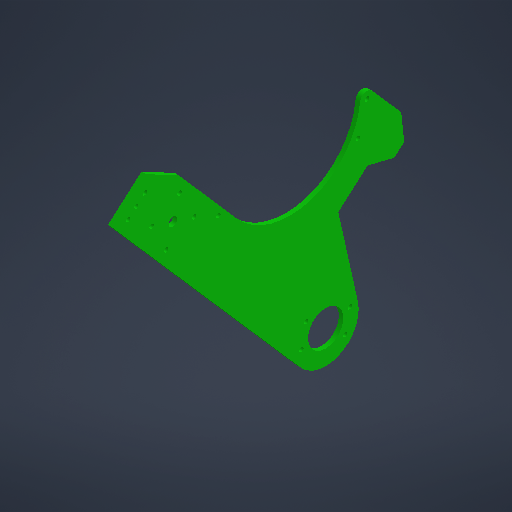
# Autodesk Inventor part: CHAPA LATERAL INTAKE V2
Saved by Autodesk Inventor 2026 (Build 300175000, 175)
## iProperties
Created: 2026-06-24
Part Number: CHAPA LATERAL INTAKE V2
Material: Genérico
Document SubType Name: Modeling
Designer: DELL
Density: 1 g/cm^3
Appearance: Verde escuro
Author: DELL
Autodesk Inventor part; units mm, degrees
ref_plane "YZ Plane" through (0, 0, 0) normal (1, 0, 0) x (0, 1, 0)
ref_plane "XZ Plane" through (0, 0, 0) normal (0, 1, 0) x (-1, 0, 0)
ref_plane "XY Plane" through (0, 0, 0) normal (0, 0, 1) x (1, 0, 0)
sketch "Esboço1" plane through (0, 0, 0) normal (1, 0, 0) x (0, 1, 0)
  circle A0 centre (0, 0) radius 20
  circle A1 centre (0, 0) radius 37.5
  dimension "d0" = 40
  dimension "d1" = 75
  constraints: 2 centre point, 2 coincident
  measures "d0" diameter of A0
  measures "d1" diameter of A1
extrude "Extrusão1" add sketch "Esboço1" along normal blind 5
sketch "Esboço3" plane through (5, 0, 0) normal (1, 0, 0) x (0, 0, -1)
  line L0 (154.1962, 109.7603) -> (153.014, 111.1125) projected
  line L1 (40.5387, 95.9825) -> (78.7824, 129.4199) projected
  line L2 (153.014, 111.1125) -> (-99.3237, 399.7205)
  circle A0 centre (0, 0) radius 37.5 projected
  line L3 (-28.231, -24.6832) -> (-242.5302, 220.4188)
  arc A1 (-100.8216, 158.3529) -> (38.988, 202.8563) centre (-40.5953, 211.0103) ccw
  line L4 (-100.8216, 158.3529) -> (-166.6433, 233.6357)
  line L5 (-166.6433, 233.6357) -> (-204.2865, 253.8562)
  circle A2 centre (46.9464, 202.0409) radius 2.5
  circle A3 centre (36.4428, 168.4765) radius 2.5
  arc A4 (52.969, 207.3066) -> (38.988, 202.8563) centre (46.9464, 202.0409) ccw
  line L6 (52.969, 207.3066) -> (85.8799, 169.6652)
  line L7 (85.8799, 169.6652) -> (14.3612, 107.1346)
  line L8 (14.3612, 107.1346) -> (36.5877, 8.2215)
  circle A5 centre (-224.6099, 219.2172) radius 2.5
  circle A6 centre (-205.4881, 235.936) radius 2.5
  circle A7 centre (-215.049, 227.5766) radius 2.5
  line L9 (-242.5302, 220.4188) -> (-204.2865, 253.8562)
  dimension "d5" = 160
  dimension "d10" = 100
  dimension "d11" = 5
  dimension "d12" = 5
  dimension "d13" = 88
  dimension "d14" = 88
  dimension "d15" = 20
  dimension "d16" = 50
  dimension "d18" = 50
  dimension "d19" = 95
  dimension "d20" = 5
  dimension "d21" = 5
  dimension "d22" = 5
  dimension "d23" = 12.7
  dimension "d25" = 12.7
  dimension "d30" = 280
  dimension "d31" = 140
  dimension "d32" = 12.7
  dimension "d33" = 12.7
  dimension "d34" = 12.7
  dimension "d35" = 12.7
  constraints: 16 end point, 7 centre point, 7 point on circle, 6 tangent, 3 perpendicular, 1 coincident, 1 point on line
  measures "d5" diameter of A1
  measures "d10" distance of L4.start L4.end
  measures "d11" diameter of A2
  measures "d12" diameter of A3
  measures "d13" distance of A1.centre A2.centre
  measures "d14" distance of A1.centre A3.centre
  measures "d15" distance from line of L2 A2.centre
  measures "d16" distance from line of L2 A3.centre
  measures "d18" distance of L6.start L6.end
  measures "d19" distance of L6.end L7.end
  measures "d20" diameter of A5
  measures "d21" diameter of A6
  measures "d22" diameter of A7
  measures "d23" distance of A5.centre A7.centre
  measures "d25" distance of A6.centre A7.centre
  measures "d30" distance between parallel lines of L1 L9
  measures "d31" distance from line of L9 A1.centre
  measures "d32" distance from line of L9 A5.centre
  measures "d33" distance from line of L9 A7.centre
  measures "d34" distance from line of L9 A6.centre
  measures "d35" distance from line of L3 A5.centre
extrude "Extrusão2" add sketch "Esboço3" against normal blind 5 contours A0 L3 L9 L5 L4 A1 A4 L6 L7 L8
sketch "Esboço4" plane through (5, 0, 0) normal (1, 0, 0) x (0, 0, -1)
  line L0 (154.1962, 109.7603) -> (153.014, 111.1125) projected
  line L1 (153.014, 111.1125) -> (-112.9577, 415.3142)
  circle A0 centre (-34.8401, 212.0241) radius 75
  circle A1 centre (-121.7601, 171.9256) radius 20
  line L2 (-204.2865, 253.8562) -> (-242.5302, 220.4188) projected
  line L3 (-242.5302, 220.4188) -> (-28.231, -24.6832) projected
  circle A2 centre (-121.7601, 171.9256) radius 2.5
  circle A3 centre (-173.5863, 191.7005) radius 5
  circle A4 centre (-22.3357, 17.5375) radius 2.5 projected
  circle A5 centre (-27.4315, -7.3461) radius 2.5 projected
  circle A6 centre (22.3357, -17.5375) radius 2.5 projected
  circle A7 centre (27.4315, 7.3461) radius 2.5 projected
  point P0 (0, 0)
  dimension "d38" = 150
  dimension "d39" = 40
  dimension "d40" = 116
  dimension "d41" = 59
  dimension "d42" = 5
  dimension "d43" = 10
  dimension "d45" = 33
  dimension "d46" = 67
  constraints: 4 centre point, 2 end point, 1 coincident, 1 tangent, 1 other
  measures "d38" diameter of A0
  measures "d39" diameter of A1
  measures "d40" distance from line of L2 A1.centre
  measures "d41" distance from line of L3 A1.centre
  measures "d42" diameter of A2
  measures "d43" diameter of A3
  measures "d45" distance from line of L3 A3.centre
  measures "d46" distance from line of L2 A3.centre
extrude "Extrusão3" cut sketch "Esboço4" against normal blind 5 contours A2 | A3 | A4 | A5 | A6 | A7
sketch "Esboço5" plane through (5, 0, 0) normal (1, 0, 0) x (0, 0, -1)
  circle A0 centre (-166.0206, 215.9476) radius 2.5193 construction
  circle A1 centre (-197.8334, 199.2662) radius 2.5193
  circle A2 centre (-149.3392, 184.1348) radius 2.5193
  circle A3 centre (-166.0206, 215.9476) radius 2.5193
  circle A4 centre (-181.152, 167.4534) radius 2.5193
  point P0 (0, 0)
  constraints: 5 centre point
extrude "Extrusão4" cut sketch "Esboço5" against normal blind 10
sketch "Esboço6" plane through (5, 0, 0) normal (1, 0, 0) x (0, 0, -1)
  line L0 (78.9782, 129.7261) -> (84.3768, 134.4529)
  line L1 (85.8799, 169.6652) -> (14.3612, 107.1346) projected
  line L2 (89.2225, 138.7154) -> (85.8799, 169.6652)
  line L3 (77.937, 128.8343) -> (47.698, 136.2818)
  line L4 (77.937, 128.8343) -> (89.2225, 138.7154)
  point P0 (0, 0)
  dimension "d58" = 55
  dimension "d61" = 15
  dimension "d62" = 25.5
  dimension "d64" = 55
  constraints: 8 end point, 1 parallel, 1 point on line, 3 other
  measures "d58" angle of L1 L2
  measures "d61" distance of L3.start L2.start
  measures "d62" distance from line of L1 L2.start
  measures "d64" angle of L1 L3
extrude "Extrusão5" add sketch "Esboço6" against normal blind 5
equation "\"d25\" = d23"
equation "\"d64\" = d58"
